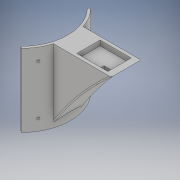
# Autodesk Inventor part: bottom camera cover
Saved by Autodesk Inventor 2017 (Build 210142000, 142)
## iProperties
Created: 2016-11-05
Part Number: bottom camera cover
Material: Generic
Document SubType Name: Modeling
Designer: Juan Maldonado
Density: 1 g/cm^3
Appearance: Default
Author: Juan Maldonado
Autodesk Inventor part; units mm, degrees
sketch "Sketch1" plane through (0, 0, 0) normal (0, 0, 1) x (1, 0, 0)
  line L0 (0, 0) -> (149.987, 0)
  line L1 (0, 0) -> (0, 177.8)
  arc A0 (0, 177.8) -> (149.987, 0) centre (690.9744, 608.5239) ccw
  dimension "d1" = 177.8
  dimension "d49" = 149.987
  constraints: 4 end point, 2 point on circle, 1 centre point, 1 horizontal, 1 vertical
  measures "d1" distance of L0.start L1.end
  measures "d49" distance of L0.end L0.start
extrude "Extrusion1" add sketch "Sketch1" along normal blind 76.2
sketch "Sketch2" plane through (0, 0, 0) normal (0, -1, 0) x (1, 0, 0)
  line L0 (53.1457, 68.072) -> (133.1457, 68.072)
  line L1 (133.1457, 68.072) -> (133.1457, 8.072)
  line L2 (133.1457, 8.072) -> (53.1457, 8.072)
  line L3 (53.1457, 8.072) -> (53.1457, 68.072)
  line L4 (0, 76.2) -> (149.987, 76.2) projected
  line L5 (0, 0) -> (149.987, 0) projected
  line L6 (149.987, 0) -> (149.987, 76.2) projected
  line L7 (0, 0) -> (0, 76.2) projected
  dimension "d46" = 80
  dimension "d47" = 60
  dimension "d48" = 8.128
  constraints: 8 end point, 2 parallel, 1 horizontal, 1 perpendicular
  measures "d46" distance of L1.end L2.end
  measures "d47" distance of L1.end L0.end
  measures "d48" distance between parallel lines of L4 L0
extrude "Extrusion2" cut sketch "Sketch2" against normal blind 12.7 contours L0 L1 L2 L3
sketch "Sketch7" plane through (0, 12.7, 0) normal (0, -1, 0) x (1, 0, 0)
  line L0 (133.1457, 8.0693) -> (133.1457, 68.072)
  line L1 (133.1457, 8.0693) -> (102.7999, 8.0693)
  line L2 (102.7999, 8.0693) -> (102.7999, 28.5329)
  line L3 (102.7999, 28.5329) -> (133.1457, 28.5329)
  line L4 (133.1457, 28.5329) -> (133.1457, 8.0693)
  point P0 (0, 0)
  point P1 (114.8738, 68.072)
  constraints: 10 end point, 2 parallel, 1 horizontal, 1 perpendicular
extrude "Extrusion5" cut sketch "Sketch7" against normal blind 50.8
shell "Shell2" thickness 2.54 removed faces 1 at (0, 118.5333, 25.4)
ref_plane "Work Plane2" through (0, 0, 0) normal (0, -1, 0) x (1, 0, 0)
sketch "Sketch8" plane through (0, 0, 0) normal (0, -1, 0) x (1, 0, 0)
  arc A0 (-29.6532, -51.665) -> (-29.6532, 126.8755) centre (-119.9849, 37.6052) ccw
  arc A1 (-34.6446, -47.6793) -> (-34.6446, 122.8898) centre (-119.9849, 37.6052) ccw
  line L0 (-34.6446, -47.6793) -> (-29.6532, -51.665)
  line L1 (-29.6532, 126.8755) -> (-34.6446, 122.8898)
  point P0 (0, 0)
  dimension "d51" = 254
  dimension "d52" = 241.3
  constraints: 4 end point, 4 point on circle, 2 centre point, 1 coincident
  measures "d51" diameter of A0
  measures "d52" diameter of A1
extrude "Extrusion6" add sketch "Sketch8" against normal blind 187.325
fillet "Fillet3" radius 3.175 2 edges at (69.4146, 82.5657, 0) (69.2254, 82.7893, 76.2)
ref_plane "Work Plane3" through (1.3198, 0, 0) normal (0.9551556, 0, -0.2961043) x (0, 1, 0)
sketch "Sketch9" plane through (1.3198, 0, 0) normal (0.9551556, 0, -0.2961043) x (0, 1, 0)
  circle A0 centre (31.2953, -29.3463) radius 3.175
  circle A1 centre (158.6554, -29.3463) radius 3.175
  point P0 (0, -0.3908)
  dimension "d56" = 6.35
  dimension "d57" = 6.35
  constraints: 2 centre point
  measures "d56" diameter of A0
  measures "d57" diameter of A1
hole "Hole3" at (-7.3697, 31.2953, -28.0303) at (-7.3697, 158.6554, -28.0303) direction (-0.9551556, 0, 0.2961043) diameter 6.35 end through all
ref_plane "Work Plane4" through (1.0087, 0, 76.2) normal (0.9527053, 0, 0.3038957) x (0, 1, 0)
sketch "Sketch10" plane through (1.0087, 0, 76.2) normal (0.9527053, 0, 0.3038957) x (0, 1, 0)
  circle A0 centre (158.9053, 27.6204) radius 3.175
  circle A1 centre (28.1971, 27.6204) radius 3.175
  point P0 (0, -72.2896)
  dimension "d65" = 6.35
  dimension "d66" = 6.35
  constraints: 2 centre point
  measures "d65" diameter of A0
  measures "d66" diameter of A1
hole "Hole4" at (-7.3851, 28.1971, 102.5141) at (-7.3851, 158.9053, 102.5141) direction (-0.9527053, 0, -0.3038957) diameter 6.35 end through all
body "Solid1"
